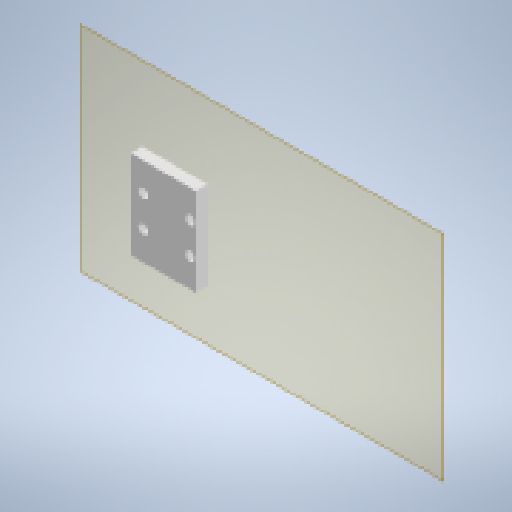
# Autodesk Inventor part: проставк
Saved by Autodesk Inventor 2024.2 (Build 282272000, 272)
## iProperties
Created: 2025-12-30
Part Number: проставк
Material: Типовые
Document SubType Name: Modeling
Designer: katya_notebook
Density: 1 g/cm^3
Appearance: По умолчанию
Author: katya_notebook
Autodesk Inventor part; units mm, degrees
ref_plane "YZ Plane" through (0, 0, 0) normal (1, 0, 0) x (0, 1, 0)
ref_plane "XZ Plane" through (0, 0, 0) normal (0, 1, 0) x (-1, 0, 0)
ref_plane "XY Plane" through (0, 0, 0) normal (0, 0, 1) x (1, 0, 0)
ref_plane "РабПлоскость1" through (51.8181, -3.2568, 14.8616) normal (0, 0, 1) x (1, 0, 0)
sketch "Эскиз1" plane through (51.8181, -3.2568, 14.8616) normal (0, 0, 1) x (1, 0, 0)
  line L0 (-26.6721, 3.7827) -> (-26.6721, -9.7173)
  line L1 (-30.7721, 8.2755) -> (-13.9721, 8.2755)
  line L2 (-13.9721, 8.2755) -> (-13.9721, -14.4178)
  line L3 (-13.9721, -14.4178) -> (-30.7721, -14.4178)
  line L4 (-30.7721, -14.4178) -> (-30.7721, 8.2755)
  point P0 (-51.8181, 3.2568)
  constraints: 10 end point, 2 parallel, 1 horizontal, 1 perpendicular, 1 vertical, 2 other
extrude "Выдавливание1" add sketch "Эскиз1" along normal blind 3
sketch "Эскиз2" plane through (51.8181, -3.2568, 14.8616) normal (0, 0, -1) x (-1, 0, 0)
  circle A0 centre (27.4758, 1.0327) radius 1.2
  circle A1 centre (15.4758, 1.0327) radius 1.2
  circle A2 centre (15.4758, -6.9673) radius 1.2
  circle A3 centre (27.4758, -6.9673) radius 1.2
  point P0 (51.8181, 3.2568)
  constraints: 4 centre point
extrude "Выдавливание2" cut sketch "Эскиз2" against normal blind 10
